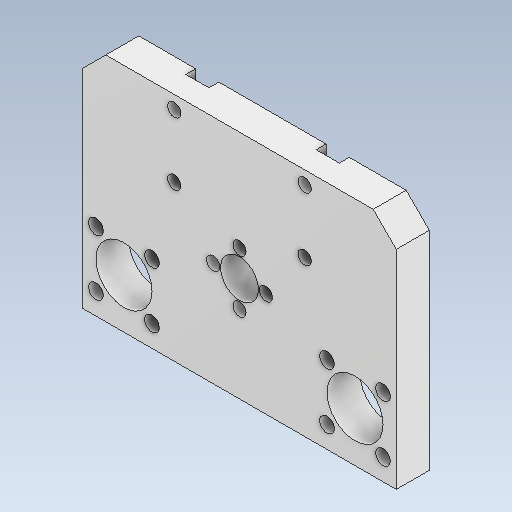
# Autodesk Inventor part: 0008-10-001
Saved by Autodesk Inventor 2020 (Build 240168000, 168)
## iProperties
Created: 2021-02-20
Part Number: 0008-10-001
Material: ABS Plastic
Document SubType Name: Modeling
Designer: Iulian Bors
Density: 1.06 g/cm^3
Appearance: Smooth - White
Mass: 61.7773 g
Surface Area: 186.476 cm^2
Volume: 58.2805 cm^3
Description: Actionator seringa
Sheet Metal Rule: Default
Author: Iulian Bors
Subject: 001
Autodesk Inventor part; units mm, degrees
ref_plane "YZ Plane" through (0, 0, 0) normal (1, 0, 0) x (0, 1, 0)
ref_plane "XZ Plane" through (0, 0, 0) normal (0, 1, 0) x (-1, 0, 0)
ref_plane "XY Plane" through (0, 0, 0) normal (0, 0, 1) x (1, 0, 0)
sketch "Sketch1" plane through (0, 0, 0) normal (0, 0, 1) x (1, 0, 0)
  line L0 (-47.5, 35) -> (47.5, 35)
  line L1 (47.5, 35) -> (47.5, -35)
  line L2 (47.5, -35) -> (-47.5, -35)
  line L3 (-47.5, -35) -> (-47.5, 35)
  point P0 (0, 0)
  point P1 (0, 35)
  point P2 (-47.5, 0)
  dimension "d0" = 95
  dimension "d1" = 70
  constraints: 8 end point, 2 midpoint, 2 parallel, 1 horizontal, 1 horizontal alignment, 1 perpendicular, 1 vertical alignment
  measures "d0" distance of L0.start L0.end
  measures "d1" distance of L0.end L1.end
extrude "Extrusion1" add sketch "Sketch1" along normal blind 10
sketch "Sketch2" plane through (0, 0, 0) normal (0, 0, -1) x (-1, 0, 0)
  line L0 (0, 71.7114) -> (0, -41.7697) construction
  line L1 (-47.5, 35) -> (47.5, 35) construction
  line L2 (-22.5, 19.157) -> (-23.5, 19.157) projected
  circle A0 centre (35, -20) radius 8.5
  line L3 (47.5, -35) -> (-47.5, -35) projected
  line L4 (-47.5, -35) -> (-47.5, 35) projected
  circle A1 centre (43.4853, -28.4853) radius 2.25
  line L5 (47.5, 35) -> (47.5, -35) construction
  line L6 (26.5147, -11.5147) -> (43.4853, -11.5147) construction
  line L7 (43.4853, -11.5147) -> (43.4853, -28.4853) construction
  line L8 (43.4853, -28.4853) -> (26.5147, -28.4853) construction
  line L9 (26.5147, -28.4853) -> (26.5147, -11.5147) construction
  circle A2 centre (43.4853, -11.5147) radius 2.25
  circle A3 centre (26.5147, -11.5147) radius 2.25
  circle A4 centre (26.5147, -28.4853) radius 2.25
  circle A5 centre (-35, -20) radius 8.5
  circle A6 centre (-43.4853, -28.4853) radius 2.25
  circle A7 centre (-43.4853, -11.5147) radius 2.25
  circle A8 centre (-26.5147, -11.5147) radius 2.25
  circle A9 centre (-26.5147, -28.4853) radius 2.25
  point P0 (0, 0)
  point P1 (0, 14.9709)
  point P2 (0, 35)
  point P3 (35, -11.5147)
  point P4 (26.5147, -20)
  dimension "d21" = 15
  dimension "d22" = 12.5
  dimension "d23" = 17
  dimension "d26" = 4.5
  dimension "d27" = 16.9706
  dimension "d28" = 16.9706
  constraints: 10 centre point, 10 end point, 5 symmetric about line, 4 coincident, 4 midpoint, 3 equal radius, 2 parallel, 2 perpendicular, 2 vertical alignment, 1 horizontal, 1 horizontal alignment, 5 other
  measures "d21" distance from line of L3 A0.centre
  measures "d22" distance from line of L5 A0.centre
  measures "d23" diameter of A0
  measures "d26" diameter of A1
  measures "d27" distance of L6.end L7.end
  measures "d28" distance of L7.end L8.end
extrude "Extrusion2" cut sketch "Sketch2" against normal through all
sketch "Sketch3" plane through (0, 0, 0) normal (0, 0, -1) x (-1, 0, 0)
  circle A0 centre (0, -3.4021) radius 5.75
  circle A1 centre (35, -20) radius 8.5 projected
  line L0 (-47.5, 35) -> (47.5, 35) projected
  line L1 (47.5, 35) -> (47.5, -35) projected
  line L2 (47.5, -35) -> (-47.5, -35) projected
  line L3 (-47.5, -35) -> (-47.5, 35) projected
  circle A2 centre (35, -20) radius 8.5 projected
  circle A3 centre (0, 4.5979) radius 2
  circle A4 centre (-8, -3.4021) radius 2
  circle A5 centre (0, -11.4021) radius 2
  circle A6 centre (8, -3.4021) radius 2
  circle A7 centre (26.5147, -11.5147) radius 2.25 projected
  circle A8 centre (-43.4853, -28.4853) radius 2.25 projected
  circle A9 centre (-43.4853, -11.5147) radius 2.25 projected
  circle A10 centre (26.5147, -28.4853) radius 2.25 projected
  circle A11 centre (43.4853, -11.5147) radius 2.25 projected
  circle A12 centre (-26.5147, -28.4853) radius 2.25 projected
  circle A13 centre (-26.5147, -11.5147) radius 2.25 projected
  circle A14 centre (43.4853, -28.4853) radius 2.25 projected
  circle A15 centre (26.5147, -11.5147) radius 2.25 projected
  circle A16 centre (-43.4853, -28.4853) radius 2.25 projected
  circle A17 centre (-43.4853, -11.5147) radius 2.25 projected
  circle A18 centre (26.5147, -28.4853) radius 2.25 projected
  circle A19 centre (43.4853, -11.5147) radius 2.25 projected
  circle A20 centre (-26.5147, -28.4853) radius 2.25 projected
  circle A21 centre (-26.5147, -11.5147) radius 2.25 projected
  circle A22 centre (43.4853, -28.4853) radius 2.25 projected
  circle A23 centre (-35, -20) radius 8.5 projected
  circle A24 centre (-35, -20) radius 8.5 projected
  line L4 (-47.5, 35) -> (47.5, 35) projected
  line L5 (47.5, 35) -> (47.5, -35) projected
  line L6 (47.5, -35) -> (-47.5, -35) projected
  line L7 (-47.5, -35) -> (-47.5, 35) projected
  point P0 (0, 0)
  point P1 (1.1874, 2.9885)
  point P2 (-1.1874, 2.9885)
  point P3 (0, -3.4021)
  point P4 (0, -35)
  dimension "d10" = 31.5979
  dimension "d12" = 11.5
  dimension "d13" = 4
  dimension "d14" = 8
  dimension "d19" = 360
  constraints: 5 centre point, 2 vertical alignment, 1 midpoint, 9 other
  measures "d10" distance from line of L2 A0.centre
  measures "d12" diameter of A0
  measures "d13" diameter of A3
  measures "d14" distance of A0.centre A3.centre
extrude "Extrusion3" cut sketch "Sketch3" against normal through all contours A0 | A3 | A4 | A5 | A6
sketch "Sketch5" plane through (0, 0, 0) normal (0, 0, -1) x (-1, 0, 0)
  circle A0 centre (19.75, 31) radius 2
  circle A1 centre (19.75, 12) radius 2
  line L0 (47.5, 35) -> (47.5, -35) projected
  line L1 (-47.5, 35) -> (47.5, 35) projected
  point P0 (0, 0)
  dimension "d29" = 27.75
  dimension "d30" = 4
  dimension "d31" = 4
  dimension "d32" = 19
  constraints: 2 centre point, 1 equal radius, 1 vertical alignment
  measures "d29" distance from line of A0.centre L0
  measures "d30" distance from line of L1 A0.centre
  measures "d31" diameter of A0
  measures "d32" distance of A0.centre A1.centre
hole "Hole1" at (-19.75, 12, 0) at (-19.75, 31, 0) direction (0, 0, 1) diameter 4 depth 11 tip angle 118 counterbore diameter 7 counterbore depth 3
sketch "Sketch6" plane through (0, 0, 0) normal (0, 0, -1) x (-1, 0, 0)
  line L0 (23.25, 27.5) -> (16.25, 27.5)
  line L1 (16.25, 27.5) -> (16.25, 35)
  line L2 (16.25, 35) -> (23.25, 35)
  line L3 (23.25, 35) -> (23.25, 27.5)
  line L4 (-47.5, 35) -> (47.5, 35) projected
  circle A0 centre (19.75, 31) radius 3.5 projected
  point P0 (0, 0)
  point P1 (16.25, 31)
  point P2 (23.25, 31)
  constraints: 8 end point, 3 tangent, 2 parallel, 1 collinear, 1 horizontal, 1 perpendicular
extrude "Extrusion4" cut sketch "Sketch6" against normal up to surface (3 mm away) contours A0 L1 L2 L3
mirror "Mirror1" about plane through (0, 0, 0) normal (1, 0, 0) of "Extrusion4", "Hole1"
chamfer "Chamfer1" distance 7 angle 45 2 edges at (-47.5, 35, 5) (47.5, 35, 5)
equation "\"BendRadius\" = Thickness"
equation "\"BendReliefWidth\" = Thickness"
equation "\"BendReliefDepth\" = 0.5 * Thickness"
equation "\"CornerReliefSize\" = 4 * Thickness"
equation "\"MinimumRemnant\" = 2 * Thickness"
equation "\"TransitionRadius\" = BendRadius"
equation "\"JacobiRadiusSize\" = Thickness"
equation "\"GapSize\" = Thickness"
equation "\"Thickness\" = 0.5"
body "Solid1"
